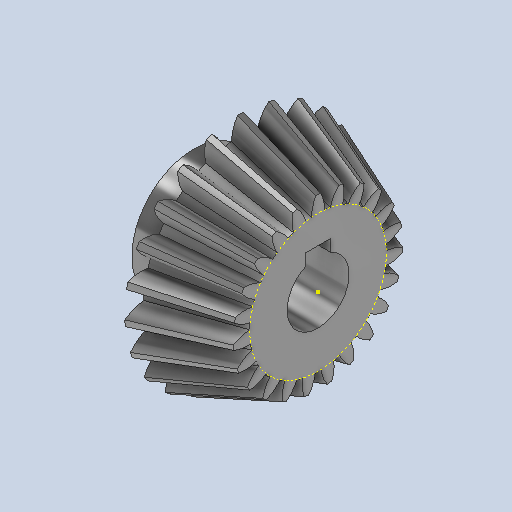
# Autodesk Inventor part: Bavel gear
Saved by Autodesk Inventor 2024 (Build 280153000, 153)
## iProperties
Created: 2023-01-01
Part Number: Bavel gear
Material: Lead
Document SubType Name: Modeling
Designer: saico
Density: 11.34 g/cm^3
Appearance: Chrome - Polished Black
Author: saico
Autodesk Inventor part; units mm, degrees
ref_plane "YZ Plane" through (0, 0, 0) normal (1, 0, 0) x (0, 1, 0)
ref_plane "XZ Plane" through (0, 0, 0) normal (0, 1, 0) x (-1, 0, 0)
ref_plane "XY Plane" through (0, 0, 0) normal (0, 0, 1) x (1, 0, 0)
sketch "Sketch1" plane through (0, 0, 0) normal (0, 0, 1) x (1, 0, 0)
  line L0 (0, 0) -> (276.3223, 0)
  line L1 (0, 0) -> (0, 20)
  line L2 (0, 20) -> (13, 20)
  line L3 (15, 22) -> (15, 31.16)
  line L4 (15, 31.16) -> (100.6114, 0)
  arc A0 (13, 20) -> (15, 22) centre (13, 22) ccw
  line L5 (40, 22.0607) -> (40, 0)
  line L6 (0, 10) -> (40, 10)
  point P0 (15, 20)
  dimension "d0" = 40
  dimension "d1" = 15
  dimension "d2" = 62.32
  dimension "d3" = 20
  dimension "d4" = 2
  dimension "d5" = 25
  dimension "d6" = 20
  constraints: 14 end point, 6 point on line, 3 perpendicular, 2 horizontal, 2 point on circle, 2 tangent, 1 centre point, 1 midpoint, 1 vertical
  measures "d0" diameter of L2 L0
  measures "d1" distance of L1.end point (15, 20)
  measures "d2" diameter of L3.end L0
  measures "d3" angle of L4 L0
  measures "d4" radius of A0
  measures "d5" distance between parallel lines of L5 L3
  measures "d6" diameter of L6 L0
revolve "Revolution1" add sketch "Sketch1" angle 360 about axis through (0, 0, 0) along (1, 0, 0) contours L1 L2 A0 L3 L4 L5 L6
sketch "Sketch2" plane through (40, 0, 0) normal (1, 0, 0) x (0, 0, -1)
  circle A0 centre (0, 0) radius 22.0607 construction
sketch "Sketch3" plane through (40, 0, 0) normal (1, 0, 0) x (0, 0, -1)
  circle A0 centre (0, 0) radius 22.0607 construction
  arc A1 (2.08, 21.9625) -> (-2.08, 21.9625) centre (0, 0) ccw
  arc A2 (0.745, 27.3148) -> (-0.745, 27.3148) centre (0, 0) ccw
  arc A3 (-0.745, 27.3148) -> (-2.08, 21.9625) centre (9.1599, 22.0017) ccw
  arc A4 (2.08, 21.9625) -> (0.745, 27.3148) centre (-9.1599, 22.0017) ccw
  dimension "d10" = 4.16
  dimension "d14" = 1.49
  dimension "d16" = 11.24
  dimension "d17" = 11.24
  constraints: 10 point on circle, 4 centre point, 2 coincident, 1 concentric
  measures "d10" distance of A0.start A0.end
  measures "d14" distance of A2.start A2.end
  measures "d16" radius of A3
  measures "d17" radius of A4
sketch "Sketch4" plane through (15, 0, 0) normal (-1, 0, 0) x (0, 0, 1)
  circle A0 centre (0, 0) radius 31.16 construction
  arc A1 (2.915, 31.0234) -> (-2.915, 31.0234) centre (0, 0) ccw
  arc A2 (0.99, 37.2669) -> (-0.96, 37.2676) centre (0, 0) ccw
  arc A3 (-0.96, 37.2676) -> (-2.915, 31.0234) centre (9.2094, 30.6555) ccw
  arc A4 (2.915, 31.0234) -> (0.99, 37.2669) centre (-9.2108, 30.7032) ccw
  dimension "d19" = 5.83
  dimension "d22" = 1.95
  dimension "d23" = 12.13
  dimension "d24" = 12.13
  constraints: 11 point on circle, 4 centre point, 2 coincident, 1 concentric
  measures "d19" distance of A0.start A0.end
  measures "d22" distance of A2.start A2.end
  measures "d23" radius of A3
  measures "d24" radius of A4
loft "Loft1" add profiles "Sketch4", "Sketch3"
pattern_circular "Circular Pattern1" count 23 over 360 about axis through (20, 0, 0) along (1, 0, 0) of "Loft1"
sketch "Sketch5" plane through (0, 0, 0) normal (-1, 0, 0) x (0, 0, 1)
  line L0 (-4, 13) -> (4, 13)
  line L1 (4, 13) -> (4, 5.8485)
  line L2 (4, 5.8485) -> (-4, 5.8485)
  line L3 (-4, 5.8485) -> (-4, 13)
  point P0 (0, 0)
  point P1 (0, 13)
  dimension "d32" = 8
  dimension "d33" = 13
  constraints: 8 end point, 2 parallel, 1 horizontal, 1 midpoint, 1 perpendicular, 1 vertical alignment
  measures "d32" distance of L0.start L0.end
  measures "d33" vertical distance of point (0, 0) L0.start
extrude "Extrusion1" cut sketch "Sketch5" against normal through all
sketch "Sketch6" plane through (15, 30.6555, 9.2094) normal (-1, 0, 0) x (0, -0.2987847, 0.9543206)
  point P0 (0.3707, -32.0069)
sketch "Sketch7" plane through (0, 0, 0) normal (-1, 0, 0) x (0, 0, 1)
  point P0 (0, 0)
  point P1 (0, 0)
  constraints: 1 coincident
body "Solid1"
